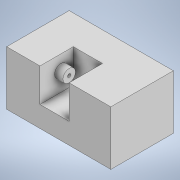
# Autodesk Inventor part: Torno
Saved by Autodesk Inventor 2021 (Build 250183000, 183)
## iProperties
Created: 2022-01-26
Part Number: Torno
Material: Genérico
Document SubType Name: Modeling
Designer: pc
Density: 1 g/cm^3
Appearance: Valor por defecto
Author: pc
Autodesk Inventor part; units mm, degrees
ref_plane "YZ Plane" through (0, 0, 0) normal (1, 0, 0) x (0, 1, 0)
ref_plane "XZ Plane" through (0, 0, 0) normal (0, 1, 0) x (-1, 0, 0)
ref_plane "XY Plane" through (0, 0, 0) normal (0, 0, 1) x (1, 0, 0)
sketch "Boceto1" plane through (0, 0, 0) normal (0, 0, 1) x (1, 0, 0)
  line L0 (0, 0) -> (2500, 0)
  line L1 (2500, 0) -> (2500, 1300)
  line L2 (2500, 1300) -> (0, 1300)
  line L3 (0, 1300) -> (0, 0)
  dimension "d0" = 2500
  dimension "d1" = 1300
  constraints: 8 end point, 2 parallel, 1 horizontal, 1 perpendicular
  measures "d0" distance of L2.end L1.end
  measures "d1" distance of L1.end L0.end
extrude "Extrusión1" add sketch "Boceto1" against normal blind 1500
sketch "Boceto2" plane through (0, 0, 0) normal (0, 0, 1) x (1, 0, 0)
  line L0 (800, 1300) -> (800, 500)
  line L1 (800, 500) -> (1500, 500)
  line L2 (1500, 500) -> (1500, 1300)
  line L3 (1500, 1300) -> (800, 1300)
  line L4 (0, 1300) -> (2500, 1300) projected
  point P0 (0, 0)
  dimension "d4" = 800
  dimension "d5" = 800
  dimension "d6" = 700
  constraints: 8 end point, 2 perpendicular, 1 collinear
  measures "d4" distance of L4.start L0.start
  measures "d5" distance of L0.start L0.end
  measures "d6" distance of L0.end L1.end
extrude "Extrusión2" cut sketch "Boceto2" against normal blind 800
sketch "Boceto3" plane through (800, 500, 0) normal (1, 0, 0) x (0, 0, -1)
  circle A0 centre (500, 450) radius 150
  line L0 (0, 0) -> (0, 800) projected
  line L1 (0, 0) -> (800, 0) projected
  point P0 (0, -500)
  dimension "d9" = 300
  dimension "d10" = 500
  dimension "d11" = 450
  constraints: 1 centre point
  measures "d9" diameter of A0
  measures "d10" distance from line of L0 A0.centre
  measures "d11" distance from line of L1 A0.centre
extrude "Extrusión3" add sketch "Boceto3" along normal blind 200
sketch "Boceto4" plane through (1000, 950, -500) normal (1, 0, 0) x (0, 0, -1)
  circle A0 centre (0, 0) radius 40
  point P0 (-500, -950)
  dimension "d14" = 80
  constraints: 1 centre point
  measures "d14" diameter of A0
extrude "Extrusión4" cut sketch "Boceto4" against normal blind 200
